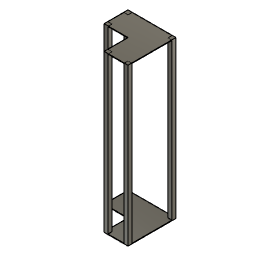
_FrameModel.d2153430-140b-4d8b-a2cd-18f9dffc3640 (Autodesk Fusion 360 design; units mm, degrees)
Autodesk Fusion 360 part; units mm, degrees
sketch "Sketch1" plane through (0, 0, 0) normal (0, 0, 1) x (1, 0, 0)
  line L0 (0, 0) -> (0, -609.6)
  line L1 (0, -609.6) -> (-304.8, -609.6)
  line L2 (-304.8, -609.6) -> (-304.8, -304.8)
  line L3 (-304.8, -304.8) -> (-609.6, -304.8)
  line L4 (-609.6, -304.8) -> (-609.6, 0)
  line L5 (-609.6, 0) -> (0, 0)
  line L6 (-403.5828, -304.8) -> (-304.8, -403.5828) construction
  line L7 (-354.1914, -354.1914) -> (0, 0) construction
  dimension "d1" = 609.6
  dimension "d2" = 609.6
  dimension "d3" = 304.8
  dimension "d4" = 304.8
  dimension "d17" = 135
  dimension "d18" = 139.7
  constraint coincident L0.start L5.end
  constraint vertical L0
  constraint perpendicular L0 L1
  constraint perpendicular L1 L2
  constraint perpendicular L2 L3
  constraint perpendicular L1 L4
  constraint perpendicular L0 L5
  constraint coincident L3 L6.start
  constraint coincident L2 L6.end
  constraint midpoint L6 L7.start
  measures "d1" distance of L0.start L0.end
  measures "d2" distance of L4.end L0.start
  measures "d3" distance of L0.end L1.end
  measures "d4" distance of L3.end L4.end
  measures "d17" angle of L2 L6
  measures "d18" distance of L6.start L6.end
extrude "Extrude1" add sketch "Sketch1" along normal blind 6.35
sketch "Sketch2" plane through (0, 0, 6.35) normal (0, 0, 1) x (-1, 0, 0)
  line L0 (609.6, 0) -> (609.6, 304.8)
  line L1 (609.6, 304.8) -> (304.8, 304.8)
  line L2 (304.8, 304.8) -> (304.8, 609.6)
  line L3 (304.8, 609.6) -> (0, 609.6)
  line L4 (0, 609.6) -> (0, 0)
  line L5 (0, 0) -> (609.6, 0)
  line L6 (304.8, 609.6) -> (254, 609.6)
  line L7 (254, 609.6) -> (254, 558.8)
  line L8 (254, 558.8) -> (304.8, 558.8)
  line L9 (304.8, 558.8) -> (304.8, 609.6)
  line L10 (0, 609.6) -> (50.8, 609.6)
  line L11 (50.8, 609.6) -> (50.8, 558.8)
  line L12 (50.8, 558.8) -> (0, 558.8)
  line L13 (0, 558.8) -> (0, 609.6)
  line L14 (0, 0) -> (50.8, 0)
  line L15 (50.8, 0) -> (50.8, 50.8)
  line L16 (50.8, 50.8) -> (0, 50.8)
  line L17 (0, 50.8) -> (0, 0)
  line L18 (609.6, 0) -> (558.8, 0)
  line L19 (558.8, 0) -> (558.8, 50.8)
  line L20 (558.8, 50.8) -> (609.6, 50.8)
  line L21 (609.6, 50.8) -> (609.6, 0)
  line L22 (609.6, 304.8) -> (558.8, 304.8)
  line L23 (558.8, 304.8) -> (558.8, 254)
  line L24 (558.8, 254) -> (609.6, 254)
  line L25 (609.6, 254) -> (609.6, 304.8)
  dimension "d7" = 50.8
  dimension "d8" = 50.8
  dimension "d9" = 50.8
  dimension "d10" = 50.8
  dimension "d11" = 50.8
  dimension "d12" = 50.8
  constraint horizontal L6
  constraint vertical L7
  constraint horizontal L8
  constraint vertical L9
  constraint coincident L2.end L3.start
  constraint horizontal L10
  constraint vertical L11
  constraint horizontal L12
  constraint vertical L13
  constraint coincident L3.end L4.start
  constraint horizontal L14
  constraint vertical L15
  constraint horizontal L16
  constraint vertical L17
  constraint coincident L4.end L5.start
  constraint horizontal L18
  constraint vertical L19
  constraint horizontal L20
  constraint vertical L21
  constraint coincident L0.start L5.end
  constraint horizontal L22
  constraint vertical L23
  constraint horizontal L24
  constraint vertical L25
  constraint coincident L0.end L1.start
  constraint collinear L11 L15
  constraint collinear L8 L12
  constraint collinear L19 L23
  constraint collinear L16 L20
  measures "d7" distance of L3.end L12.end
  measures "d8" distance of L3.end L10.end
  measures "d9" distance of L2.end L6.end
  measures "d10" distance of L4.end L16.end
  measures "d11" distance of L0.start L18.end
  measures "d12" distance of L0.end L24.end
extrude "Extrude2" add sketch "Sketch2" along normal blind 1981.2 contours L0 L5 L18 L19 L20 L21 | L0 L1 L22 L23 L24 L25 | L4 L5 L14 L15 L16 L17 | L3 L4 L10 L11 L12 L13 | L2 L3 L6 L7 L8 L9
sketch "Sketch3" plane through (0, 0, 1987.55) normal (0, 0, 1) x (-1, 0, 0)
  line L0 (0, 558.8) -> (50.8, 558.8)
  line L1 (50.8, 558.8) -> (50.8, 609.6)
  line L2 (50.8, 609.6) -> (0, 609.6)
  line L3 (0, 609.6) -> (0, 558.8)
  line L4 (0, 609.6) -> (0, 0)
  line L5 (0, 609.6) -> (304.8, 609.6)
  line L6 (304.8, 609.6) -> (304.8, 304.8)
  line L7 (304.8, 304.8) -> (609.6, 304.8)
  line L8 (609.6, 304.8) -> (609.6, 0)
  line L9 (609.6, 0) -> (0, 0)
  point P0 (304.8, 609.6)
  point P1 (609.6, 304.8)
  constraint coincident L2.end L3.start
  constraint coincident L4.end L9.end
  constraint perpendicular L1 L5
  constraint perpendicular L5 L6
  constraint perpendicular L6 L7
  constraint perpendicular L7 L8
  constraint perpendicular L4 L9
  constraint coincident P0 L5.end
  constraint coincident P1 L7.end
extrude "Extrude3" add sketch "Sketch3" along normal blind 6.35
